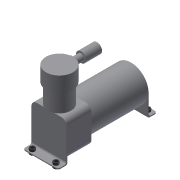
# Autodesk Inventor part: Viair Compressor
Saved by Autodesk Inventor 2013 (Build 170138000, 138)
## iProperties
Created: 2013-12-22
Part Number: Viair Compressor
Material: Generic
Document SubType Name: Modeling
Designer: Nemo
Mass: 1084.09 g
Surface Area: 434.122 cm^2
Volume: 376.751 cm^3
Density: 2.87746 g/cm^3
Author: Nemo
Autodesk Inventor part; units mm, degrees
ref_plane "YZ Plane" through (0, 0, 0) normal (1, 0, 0) x (0, 1, 0)
ref_plane "XZ Plane" through (0, 0, 0) normal (0, 1, 0) x (-1, 0, 0)
ref_plane "XY Plane" through (0, 0, 0) normal (0, 0, 1) x (1, 0, 0)
sketch "Sketch1" plane through (0, 0, 0) normal (0, 0, 1) x (1, 0, 0)
  circle A0 centre (0, 0) radius 26.797
  dimension "d0" = 53.594
  constraints: 1 centre point, 1 coincident
  measures "d0" diameter of A0
extrude "Extrusion1" add sketch "Sketch1" along normal blind 85.852
sketch "Sketch2" plane through (0, 0, 85.852) normal (0, 0, 1) x (1, 0, 0)
  circle A0 centre (0, 0) radius 26.797 projected
  line L0 (26.797, -26.797) -> (-26.797, -26.797)
  line L1 (-26.797, -26.797) -> (-26.797, 26.797)
  line L2 (-26.797, 26.797) -> (26.797, 26.797)
  line L3 (26.797, 26.797) -> (26.797, -26.797)
  line L4 (26.797, -26.797) -> (-26.797, 26.797) construction
  line L5 (-26.797, -26.797) -> (26.797, 26.797) construction
  constraints: 12 end point, 2 midpoint, 2 parallel, 1 horizontal, 1 perpendicular
extrude "Extrusion2" add sketch "Sketch2" along normal blind 38.1
sketch "Sketch3" plane through (-26.797, 26.797, 85.852) normal (0, 1, 0) x (1, 0, 0)
  circle A0 centre (26.797, -22.019) radius 17.9552
  point P0 (26.797, 0)
  point P1 (26.797, 85.852)
  dimension "d5" = 35.9104
  constraints: 1 centre point, 1 vertical alignment
  measures "d5" diameter of A0
extrude "Extrusion3" add sketch "Sketch3" along normal blind 29.083
sketch "Sketch4" plane through (0, 55.88, 107.871) normal (0, 1, 0) x (1, 0, 0)
  circle A0 centre (0, 0) radius 17.9552 construction
  circle A1 centre (0, 0) radius 20.6375
  line L0 (3.81, 20.1295) -> (-3.81, 20.1295)
  line L1 (-3.81, 20.1295) -> (-3.81, 21.1455)
  line L2 (-3.81, 21.1455) -> (3.81, 21.1455)
  line L3 (3.81, 21.1455) -> (3.81, 20.1295)
  line L4 (3.81, 20.1295) -> (-3.81, 21.1455) construction
  line L5 (-3.81, 20.1295) -> (3.81, 21.1455) construction
  point P0 (0, 107.871)
  point P1 (0, 20.6375)
  dimension "d9" = 41.275
  dimension "d10" = 7.62
  dimension "d11" = 1.016
  constraints: 12 end point, 2 midpoint, 2 parallel, 1 coincident, 1 horizontal, 1 perpendicular, 1 vertical alignment, 2 other
  measures "d10" distance of L1.end L2.end
  measures "d11" distance of L0.end L1.end
extrude "Extrusion4" add sketch "Sketch4" along normal blind 22.86
sketch "Sketch5" plane through (3.81, 55.88, 86.7255) normal (0, 0, -1) x (-1, 0, 0)
  circle A0 centre (3.81, 16.1903) radius 5.1597
  point P0 (3.81, -55.88)
  constraints: 1 centre point
extrude "Extrusion5" add sketch "Sketch5" along normal blind 11.7475
sketch "Sketch6" plane through (0, 72.0703, 74.978) normal (0, 0, -1) x (-1, 0, 0)
  circle A0 centre (0, 0) radius 5.1597 projected
  circle A1 centre (0, 0) radius 7.7593
  point P0 (0, -72.0703)
  constraints: 1 centre point, 1 coincident
extrude "Extrusion6" add sketch "Sketch6" along normal blind 24.4475 contours A0 | A1
sketch "Sketch7" plane through (0, -26.797, 85.852) normal (0, -1, 0) x (1, 0, 0)
  line L0 (26.797, 0) -> (26.797, 38.1) projected
  line L1 (-26.797, 38.1) -> (26.797, 38.1)
  line L2 (26.797, 38.1) -> (26.797, 36.576)
  line L3 (26.797, 36.576) -> (-26.797, 36.576)
  line L4 (-26.797, 36.576) -> (-26.797, 38.1)
  point P0 (0, -85.852)
  dimension "d18" = 1.524
  constraints: 8 end point, 2 parallel, 1 horizontal, 1 perpendicular, 1 point on line
  measures "d18" distance between parallel lines of L1 L3
extrude "Extrusion7" add sketch "Sketch7" along normal blind 6.35
sketch "Sketch8" plane through (0, 0, 123.952) normal (0, 0, 1) x (1, 0, 0)
  line L0 (26.797, 26.797) -> (26.797, -33.147) projected
  line L1 (-26.797, -33.147) -> (26.797, -33.147)
  line L2 (26.797, -33.147) -> (26.797, -31.623)
  line L3 (26.797, -31.623) -> (-26.797, -31.623)
  line L4 (-26.797, -31.623) -> (-26.797, -33.147)
  point P0 (0, 0)
  dimension "d22" = 1.524
  constraints: 8 end point, 2 parallel, 1 horizontal, 1 perpendicular, 1 point on line
  measures "d22" distance between parallel lines of L1 L3
extrude "Extrusion8" add sketch "Sketch8" along normal blind 12.7
fillet "Fillet1" radius 3.175 2 edges at (0, -31.623, 123.952) (0, -33.147, 122.428)
sketch "Sketch9" plane through (-26.797, -31.623, 136.652) normal (0, 1, 0) x (1, 0, 0)
  line L0 (53.594, 0) -> (0, 0) projected
  line L1 (53.594, 9.525) -> (53.594, 0) projected
  line L2 (8.763, 5.461) -> (44.831, 5.461) construction
  line L3 (0, 9.525) -> (0, 0) projected
  line L4 (0, 4.7625) -> (53.594, 4.7625) construction
  point P0 (26.797, 136.652)
  point P1 (26.797, 5.461)
  point P2 (26.797, 0)
  dimension "d27" = 36.068
  dimension "d59" = 0.6985
  constraints: 4 end point, 4 midpoint, 2 coincident, 1 perpendicular, 1 vertical alignment
  measures "d27" distance of L2.start L2.end
  measures "d59" distance between parallel lines of L4 L2
hole "Hole1" at (-18.034, -31.623, 131.191) at (18.034, -31.623, 131.191) direction (0, -1, 0) diameter 4.826 end through all
fillet "Fillet2" radius 3.175 2 edges at (26.797, -32.385, 136.652) (-26.797, -32.385, 136.652)
sketch "Sketch10" plane through (0, 0, 0) normal (0, 0, -1) x (-1, 0, 0)
  line L0 (-26.797, -28.448) -> (26.797, -28.448) projected
  line L1 (-26.797, 26.797) -> (-26.797, -28.448) projected
  line L2 (-26.797, 26.797) -> (-7.9869, 26.797) projected
  line L3 (-7.9869, 26.797) -> (7.9869, 26.797) projected
  line L4 (7.9869, 26.797) -> (26.797, 26.797) projected
  line L5 (26.797, 26.797) -> (26.797, -28.448) projected
  line L6 (-26.797, -28.448) -> (26.797, -28.448)
  line L7 (26.797, -28.448) -> (26.797, -33.147)
  line L8 (26.797, -33.147) -> (-26.797, -33.147)
  line L9 (-26.797, -33.147) -> (-26.797, -28.448)
  dimension "d39" = 4.699
  constraints: 8 end point, 2 parallel, 1 collinear, 1 horizontal, 1 perpendicular, 1 point on line
  measures "d39" distance between parallel lines of L6 L8
extrude "Extrusion9" add sketch "Sketch10" along normal blind 1.524
sketch "Sketch11" plane through (0, 0, -1.524) normal (0, 0, -1) x (-1, 0, 0)
  line L0 (26.797, -33.147) -> (26.797, 26.797) projected
  line L1 (-26.797, -33.147) -> (26.797, -33.147)
  line L2 (26.797, -33.147) -> (26.797, -31.623)
  line L3 (26.797, -31.623) -> (-26.797, -31.623)
  line L4 (-26.797, -31.623) -> (-26.797, -33.147)
  point P0 (0, 0)
  dimension "d42" = 1.524
  constraints: 8 end point, 2 parallel, 1 horizontal, 1 perpendicular, 1 point on line
  measures "d42" distance between parallel lines of L1 L3
extrude "Extrusion10" add sketch "Sketch11" along normal blind 12.7
fillet "Fillet3" radius 3.175 2 edges at (0, -33.147, 0) (0, -31.623, -1.524)
sketch "Sketch12" plane through (-26.797, -31.623, -14.224) normal (0, 1, 0) x (1, 0, 0)
  line L0 (53.594, -9.525) -> (0, -9.525) projected
  line L1 (0, -9.525) -> (0, 0) projected
  line L2 (8.763, -5.461) -> (44.831, -5.461) construction
  line L3 (53.594, -9.525) -> (53.594, 0) projected
  line L4 (0, -4.7625) -> (53.594, -4.7625) construction
  point P0 (26.797, -14.224)
  point P1 (26.797, -5.461)
  point P2 (26.797, -9.525)
  dimension "d47" = 36.068
  dimension "d57" = 0.6985
  constraints: 4 end point, 4 midpoint, 2 coincident, 1 perpendicular, 1 vertical alignment
  measures "d47" distance of L2.start L2.end
  measures "d57" distance between parallel lines of L2 L4
hole "Hole2" at (-18.034, -31.623, -8.763) at (18.034, -31.623, -8.763) direction (0, -1, 0) diameter 4.826 end through all
fillet "Fillet4" radius 3.175 2 edges at (26.797, -32.385, -14.224) (-26.797, -32.385, -14.224)
sketch "Sketch13" plane through (0, 0, 0) normal (0, 0, 1) x (1, 0, 0)
  arc A0 (26.797, 0) -> (0, 26.797) centre (0, 0) ccw projected
  line L0 (26.797, 26.797) -> (26.797, 0) projected
  line L1 (26.797, 26.797) -> (0, 26.797) projected
extrude "Extrusion11" cut sketch "Sketch13" against normal through all
sketch "Sketch14" plane through (0, 0, 0) normal (0, 0, 1) x (1, 0, 0)
  arc A0 (0, 26.797) -> (-26.797, 0) centre (0, 0) ccw projected
  line L0 (0, 26.797) -> (-26.797, 26.797) projected
  line L1 (-26.797, 0) -> (-26.797, 26.797) projected
extrude "Extrusion12" cut sketch "Sketch14" against normal through all
sketch "Sketch15" plane through (0, -33.147, 85.852) normal (0, -1, 0) x (1, 0, 0)
  circle A0 centre (-18.034, 45.339) radius 2.413 projected
  circle A1 centre (18.034, 45.339) radius 2.413 projected
  circle A2 centre (-18.034, 45.339) radius 3.9751
  circle A3 centre (18.034, 45.339) radius 3.9751
  circle A4 centre (-18.034, -94.615) radius 2.413 projected
  circle A5 centre (18.034, -94.615) radius 2.413 projected
  circle A6 centre (-18.034, -94.615) radius 3.9751
  circle A7 centre (18.034, -94.615) radius 3.9751
  point P0 (0, -85.852)
  dimension "d64" = 7.9502
  dimension "d65" = 7.9502
  dimension "d70" = 7.9502
  dimension "d71" = 7.9502
  constraints: 4 centre point, 4 coincident
  measures "d64" diameter of A2
  measures "d65" diameter of A3
  measures "d70" diameter of A6
  measures "d71" diameter of A7
extrude "Extrusion13" add sketch "Sketch15" along normal blind 3.175 and the other way blind 4.699 separate body
fillet "Fillet5" radius 8.255 4 edges at (26.797, 26.797, 104.902) (26.797, -26.797, 104.14) (-26.797, -26.797, 104.14) (-26.797, 26.797, 104.902)
body "Solid1"
body "Solid2"
